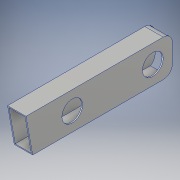
# Autodesk Inventor part: ARM_030_TopIntakeSide
Saved by Autodesk Inventor 2018.3 (Build 223284000, 284)
## iProperties
Created: 2020-02-04
Part Number: ARM_030_TopIntakeSide
Material: Aluminum 6061
Document SubType Name: Modeling
Designer: 22turnmaxw
Density: 2.7 g/cm^3
Appearance: Aluminum - Flat
Author: 22turnmaxw
Autodesk Inventor part; units mm, degrees
ref_plane "YZ Plane" through (0, 0, 0) normal (1, 0, 0) x (0, 1, 0)
ref_plane "XZ Plane" through (0, 0, 0) normal (0, 1, 0) x (-1, 0, 0)
ref_plane "XY Plane" through (0, 0, 0) normal (0, 0, 1) x (1, 0, 0)
sketch "Sketch1" plane through (0, 0, 0) normal (0, 0, 1) x (1, 0, 0)
  line L0 (0, 0) -> (25.4, 0)
  line L1 (25.4, 0) -> (25.4, 50.8)
  line L2 (25.4, 50.8) -> (0, 50.8)
  line L3 (0, 50.8) -> (0, 0)
  line L4 (1.5875, 1.5875) -> (23.8125, 1.5875)
  line L5 (23.8125, 1.5875) -> (23.8125, 49.2125)
  line L6 (23.8125, 49.2125) -> (1.5875, 49.2125)
  line L7 (1.5875, 49.2125) -> (1.5875, 1.5875)
  dimension "d0" = 25.4
  dimension "d1" = 50.8
  dimension "d2" = 1.5875
  constraints: 16 end point, 4 parallel, 2 perpendicular, 1 horizontal, 3 other
  measures "d0" distance of L1.end L2.end
  measures "d1" distance of L0.end L1.end
  measures "d2" distance between parallel lines of L3 L7
extrude "Extrusion1" add sketch "Sketch1" along normal blind 365.252
sketch "Sketch2" plane through (25.4, 0, 0) normal (1, 0, 0) x (0, 0, -1)
  line L0 (0, 50.8) -> (-365.252, 50.8) projected
  line L1 (-365.252, 50.8) -> (-356.075, 0)
  line L2 (-356.075, 0) -> (-365.252, 0)
  line L3 (0, 1.5875) -> (-365.252, 1.5875) projected
  line L4 (-365.252, 50.8) -> (-365.252, 0) projected
  line L5 (-365.252, 0) -> (-365.252, 50.8)
  point P0 (0, 0)
  dimension "d5" = 10.24
  constraints: 6 end point, 1 collinear, 1 parallel
  measures "d5" angle of L4 L1
sketch "Sketch3" plane through (25.4, 0, 0) normal (1, 0, 0) x (0, 0, -1)
  line L0 (0, 0) -> (0, 50.8) projected
  line L1 (0, 50.8) -> (-365.252, 50.8) projected
  line L2 (0, 0) -> (-365.252, 0) projected
  line L3 (-365.252, 0) -> (-365.252, 50.8) projected
  point P0 (-50.8, 25.4)
  point P1 (-190.5737, 25.4)
  point P2 (-356.075, 0)
  point P3 (-301.5742, 25.4)
  dimension "d9" = 50.8
  dimension "d10" = 25.4
  dimension "d19" = 25.4
  dimension "d21" = 25.4
  dimension "d25" = 63.6778
  dimension "d28" = 174.6783
  measures "d9" distance from line of L0 point (-50.8, 25.4)
  measures "d10" distance from line of L1 point (-50.8, 25.4)
  measures "d19" distance from line of L2 point (-190.574, 25.4)
  measures "d21" distance from line of L2 point (-301.574, 25.4)
  measures "d25" distance from line of L3 point (-301.574, 25.4)
  measures "d28" distance from line of L3 point (-190.574, 25.4)
hole "Hole1" at (25.4, 25.4, 50.8) at (25.4, 25.4, 190.5737) at (25.4, 25.4, 301.5742) direction (-1, 0, 0) diameter 22.225 depth 25.4 tip angle 118
sketch "Sketch4" plane through (25.4, 0, 0) normal (1, 0, 0) x (0, 0, -1)
  line L0 (0, 50.8) -> (-365.252, 50.8) projected
  line L1 (-163.5862, 50.8) -> (0, 50.8)
  line L2 (0, 50.8) -> (0, 0)
  line L3 (0, 0) -> (-163.5862, 0)
  line L4 (-163.5862, 0) -> (-163.5862, 50.8)
  circle A0 centre (-190.5737, 25.4) radius 11.1125 projected
  dimension "d22" = 26.9875
  constraints: 8 end point, 2 parallel, 1 horizontal, 1 perpendicular, 1 point on line
  measures "d22" distance from line of A0.centre L4
extrude "Extrusion3" cut sketch "Sketch4" against normal blind 25.4 contours L2 L3 L4 L0
extrude "Extrusion4" cut sketch "Sketch2" against normal blind 25.4
fillet "Fillet1" radius 12.7 2 edges at (12.7, 50.8, 163.5862) (12.7, 0, 163.5862)
sketch "Sketch5" plane through (25.4, 12.7, 163.5862) normal (1, 0, 0) x (0, 0, -1)
  circle A0 centre (-26.9875, 12.7) radius 11.1125 projected
  circle A1 centre (-137.988, 12.7) radius 11.1125 projected
  point P0 (163.5862, -12.7)
  dimension "d30" = 0
  dimension "d31" = 0
  constraints: 1 coincident
  measures "d30" distance of A0.centre point (-26.988, 12.7)
  measures "d31" distance of A0.centre point (-26.988, 12.7)
hole "Hole2" at (25.4, 25.4, 190.5737) at (25.4, 25.4, 301.5742) direction (-1, 0, 0) diameter 28.575 depth 1.5875 tip angle 118
body "Solid1"
